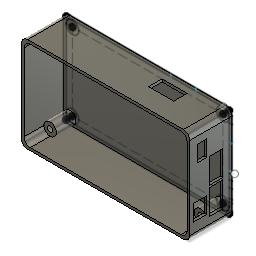
Enclosure PlayGround4Robotics v7 (Autodesk Fusion 360 design; units mm, degrees)
Autodesk Fusion 360 part; units mm, degrees
sketch "Sketch1" plane through (0, 0, 0) normal (0, 0, 1) x (1, 0, 0)
  line L0 (3.5, 0) -> (87.5, 0)
  line L1 (0, 3.5) -> (0, 46.5)
  line L2 (3.5, 50) -> (87.5, 50)
  line L3 (91, 46.5) -> (91, 3.5)
  line L4 (3.5, 0) -> (3.5, 50) construction
  line L5 (0, 3.5) -> (91, 3.5) construction
  circle A0 centre (3.5, 3.5) radius 1.5
  line L6 (87.5, 0) -> (87.5, 50) construction
  line L7 (0, 46.5) -> (91, 46.5) construction
  circle A1 centre (87.5, 3.5) radius 1.5
  circle A2 centre (87.5, 46.5) radius 1.5
  circle A3 centre (3.5, 46.5) radius 1.5
  arc A4 (3.5, 50) -> (0, 46.5) centre (3.5, 46.5) ccw
  arc A5 (91, 46.5) -> (87.5, 50) centre (87.5, 46.5) ccw
  arc A6 (0, 3.5) -> (3.5, 0) centre (3.5, 3.5) ccw
  arc A7 (87.5, 0) -> (91, 3.5) centre (87.5, 3.5) ccw
  circle A8 centre (3.5, 46.5) radius 3.5
  circle A9 centre (3.5, 3.5) radius 3.5
  circle A10 centre (87.5, 3.5) radius 3.5
  circle A11 centre (87.5, 46.5) radius 3.5
  line L8 (2, 51.5) -> (89, 51.5)
  line L9 (2, -1.5) -> (89, -1.5)
  line L10 (92.5, 2) -> (92.5, 48)
  line L11 (-1.5, 2) -> (-1.5, 48)
  arc A12 (92.5, 48) -> (89, 51.5) centre (89, 48) ccw
  arc A13 (2, 51.5) -> (-1.5, 48) centre (2, 48) ccw
  arc A14 (89, -1.5) -> (92.5, 2) centre (89, 2) ccw
  arc A15 (-1.5, 2) -> (2, -1.5) centre (2, 2) ccw
  line L12 (91, 7.5) -> (92.5, 7.5)
  line L13 (91, 16.5) -> (92.5, 16.5)
  line L14 (91, 44) -> (92.5, 44)
  line L15 (91, 35) -> (92.5, 35)
  line L16 (91, 12.7) -> (92.5, 12.7)
  line L17 (91, 19.7) -> (92.5, 19.7)
  line L18 (91, 5.7) -> (92.5, 5.7)
  line L19 (91, 34.8) -> (92.5, 34.8)
  line L20 (58.5, 50) -> (58.5, 51.5)
  line L21 (72.5, 50) -> (72.5, 51.5)
  line L22 (94, 20.8) -> (91, 20.8)
  point P0 (91, 0)
  point P1 (0, 50)
  point P2 (91, 50)
  dimension "d1" = 91
  dimension "d2" = 50
  dimension "d3" = 91
  dimension "d4" = 3.5
  dimension "d5" = 3.5
  dimension "d6" = 3
  dimension "d7" = 3.5
  dimension "d8" = 3.5
  dimension "d9" = 3
  dimension "d10" = 3
  dimension "d11" = 3
  dimension "d12" = 3.5
  dimension "d13" = 3.5
  dimension "d14" = 3.5
  dimension "d15" = 3.5
  dimension "d16" = 7
  dimension "d17" = 7
  dimension "d18" = 7
  dimension "d19" = 7
  dimension "d20" = 1.5
  dimension "d21" = 1.5
  dimension "d22" = 1.5
  dimension "d23" = 1.5
  dimension "d24" = 3.5
  dimension "d25" = 3.5
  dimension "d26" = 3.5
  dimension "d27" = 3.5
  dimension "d28" = 7.5
  dimension "d29" = 9
  dimension "d30" = 6
  dimension "d31" = 9
  dimension "d32" = 12.7
  dimension "d34" = 7
  dimension "d35" = 7
  constraint horizontal L0
  constraint perpendicular L0 L1
  constraint perpendicular L1 L2
  constraint coincident L0 L4.start
  constraint coincident L2 L4.end
  constraint perpendicular L2 L4
  constraint coincident L1 L5.start
  constraint coincident L3 L5.end
  constraint perpendicular L3 L5
  constraint coincident L5 A0.centre
  constraint coincident L4 A0.centre
  constraint coincident L0 L6.start
  constraint perpendicular L5 L6
  constraint coincident L1 L7.start
  constraint coincident L3 L7.end
  constraint perpendicular L3 L7
  constraint coincident L6 A1.centre
  constraint coincident L5 A1.centre
  constraint coincident L7 A2.centre
  constraint coincident L6 A2.centre
  constraint coincident L7 A3.centre
  constraint coincident L4 A3.centre
  constraint coincident P1 L2
  constraint tangent L2 A4
  constraint tangent L1 A4
  constraint coincident P2 L2
  constraint coincident P2 L3
  constraint tangent L2 A5
  constraint tangent L3 A5
  constraint coincident origin L1
  constraint coincident origin L0
  constraint tangent L1 A6
  constraint tangent L0 A6
  constraint coincident P0 L0
  constraint coincident P0 L3
  constraint tangent L0 A7
  constraint tangent L3 A7
  constraint concentric A3 A8
  constraint concentric A0 A9
  constraint concentric A1 A10
  constraint concentric A2 A11
  constraint parallel L7 L8
  constraint horizontal L9
  constraint perpendicular L8 L10
  constraint perpendicular L8 L11
  constraint tangent L8 A12
  constraint tangent L10 A12
  constraint tangent L11 A13
  constraint tangent L8 A13
  constraint tangent L10 A14
  constraint tangent L9 A14
  constraint tangent L11 A15
  constraint tangent L9 A15
  constraint coincident L3 L12.start
  constraint coincident L10 L12.end
  constraint perpendicular L10 L12
  constraint coincident L3 L13.start
  constraint coincident L10 L13.end
  constraint perpendicular L10 L13
  constraint coincident L3 L14.start
  constraint coincident L10 L14.end
  constraint perpendicular L10 L14
  constraint coincident L3 L15.start
  constraint coincident L10 L15.end
  constraint perpendicular L10 L15
  constraint coincident L3 L16.start
  constraint coincident L10 L16.end
  constraint perpendicular L10 L16
  constraint coincident L3 L17.start
  constraint coincident L10 L17.end
  constraint perpendicular L10 L17
  constraint coincident L3 L18.start
  constraint coincident L10 L18.end
  constraint perpendicular L10 L18
  constraint coincident L3 L19.start
  constraint coincident L10 L19.end
  constraint perpendicular L10 L19
  constraint coincident L2 L20.start
  constraint coincident L8 L20.end
  constraint perpendicular L8 L20
  constraint coincident L2 L21.start
  constraint coincident L8 L21.end
  constraint perpendicular L8 L21
  constraint coincident L3 L22.end
  constraint perpendicular L3 L22
  measures "d1" distance of origin P0
  measures "d2" distance of origin P1
  measures "d3" distance of P1 P2
  measures "d4" distance of L1 L4
  measures "d5" distance of L0 L5
  measures "d6" diameter of A0
  measures "d7" distance of L3 L6
  measures "d8" distance of L2 L7
  measures "d9" diameter of A1
  measures "d10" diameter of A2
  measures "d11" diameter of A3
  measures "d12" radius of A4
  measures "d13" radius of A5
  measures "d14" radius of A6
  measures "d15" radius of A7
  measures "d16" diameter of A8
  measures "d17" diameter of A9
  measures "d18" diameter of A10
  measures "d19" diameter of A11
  measures "d20" distance of L0 L9
  measures "d21" distance of L2 L8
  measures "d22" distance of L1 L11
  measures "d23" distance of L3 L10
  measures "d24" radius of A12
  measures "d25" radius of A13
  measures "d26" radius of A14
  measures "d27" radius of A15
  measures "d28" distance of L0 L12
  measures "d29" distance of L12 L13
  measures "d30" distance of L2 L14
  measures "d31" distance of L14 L15
  measures "d32" distance of L0 L16
  measures "d34" distance of L16 L18
  measures "d35" distance of L16.start L17
extrude "Extrude1" add sketch "Sketch1" along normal blind 1.5 contours L0 L1 L2 L3 A8 A9 A10 A11 | L0 L1 L2 L3 A4 A6 A7 A8 A9 A10 L8 L9 L10 L11 A13 A14 A15 L18 L20 | A6 A9 | A7 A10 | A4 A8 | L3 L10 L12 L18 | L3 L10 L12 L16 | L2 L8 L20 L21 | L3 L10 L13 L16 | L2 L3 A5 A11 L8 L10 A12 L14 L21 | L3 L10 L13 L17 | A5 A11 | L3 L10 L17 L22 | L3 L10 L19 L22 | L3 L10 L14 L15 | A0 | A1 | A2 | A3
extrude "Extrude2" add sketch "Sketch1" along normal blind 12.5 contours A6 A9 | A7 A10 | A4 A8 | A5 A11
extrude "Extrude3" add sketch "Sketch1" along normal blind 23.5 contours L0 L1 L2 L3 A4 A6 A7 A8 A9 A10 L8 L9 L10 L11 A13 A14 A15 L18 L20 | L3 L10 L12 L18 | L3 L10 L12 L16 | L2 L8 L20 L21 | L3 L10 L13 L16 | L2 L3 A5 A11 L8 L10 A12 L14 L21 | L3 L10 L13 L17 | L3 L10 L17 L22 | L3 L10 L19 L22 | L3 L10 L14 L15 | L3 L10 L15 L19
extrude "Extrude4" cut sketch "Sketch1" along normal blind 7.5 from surface at 5 contours L3 L10 L12 L18 | L3 L10 L12 L16 | L2 L8 L20 L21 | L3 L10 L13 L16 | L3 L10 L13 L17 | L3 L10 L19 L22
extrude "Extrude5" cut sketch "Sketch1" along normal blind 7.5 from surface at 14 contours L3 L10 L12 L16 | L3 L10 L13 L16
extrude "Extrude6" cut sketch "Sketch1" along normal blind 5 from surface at 14 contours L3 L10 L14 L15
